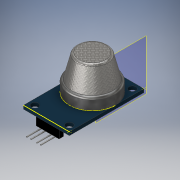
# Autodesk Inventor part: CO2_Sensor
Saved by Autodesk Inventor 2017.2 (Build 212223000, 223)
## iProperties
Created: 2017-03-02
Part Number: CO2_Sensor
Material: Generic
Document SubType Name: Modeling
Designer: prosp
Density: 1 g/cm^3
Appearance: Default
Author: prosp
Autodesk Inventor part; units mm, degrees
ref_plane "YZ Plane" through (0, 0, 0) normal (1, 0, 0) x (0, 1, 0)
ref_plane "XZ Plane" through (0, 0, 0) normal (0, 1, 0) x (-1, 0, 0)
ref_plane "XY Plane" through (0, 0, 0) normal (0, 0, 1) x (1, 0, 0)
sketch "Sketch1" plane through (0, 0, 0) normal (0, 1, 0) x (-1, 0, 0)
  line L0 (10, 16.25) -> (10, -16.25)
  line L1 (10, -16.25) -> (-10, -16.25)
  line L2 (-10, -16.25) -> (-10, 16.25)
  line L3 (-10, 16.25) -> (10, 16.25)
  line L4 (10, 16.25) -> (-10, -16.25) construction
  line L5 (10, -16.25) -> (-10, 16.25) construction
  point P0 (0, 0)
  dimension "d0" = 32.5
  dimension "d1" = 20
  constraints: 12 end point, 2 midpoint, 2 parallel, 1 perpendicular, 1 vertical
  measures "d0" distance of L0.start L0.end
  measures "d1" distance of L0.end L1.end
extrude "Extrusion1" add sketch "Sketch1" along normal blind 1.5
sketch "Sketch2" plane through (0, 1.5, 0) normal (0, 1, 0) x (1, 0, 0)
  line L0 (-10, -16.25) -> (10, -16.25) projected
  point P0 (0, 0)
sketch "Sketch3" plane through (0, 1.5, 0) normal (0, 1, 0) x (1, 0, 0)
  line L0 (-10, -16.25) -> (10, -16.25) projected
  circle A0 centre (0, 3.75) radius 10
  point P0 (0, 0)
  dimension "d7" = 20
  constraints: 1 centre point
  measures "d7" diameter of A0
extrude "Extrusion2" add sketch "Sketch3" along normal blind 5
sketch "Sketch4" plane through (0, 1.5, 0) normal (0, 1, 0) x (1, 0, 0)
  arc A0 (-10, 3.75) -> (10, 3.75) centre (0, 3.75) ccw projected
  point P0 (0, 0)
  point P1 (10, -16.25)
  point P2 (10, 16.25)
fillet "Fillet1" radius 1 1 edges at (-10, 6.5, -3.75)
ref_plane "Work Plane6" through (0, 0, -16.25) normal (-1, 0, 0) x (0, 0, 1)
sketch "Sketch8" plane through (0, 0, -16.25) normal (-1, 0, 0) x (0, 0, 1)
  line L0 (3.5, 6.5) -> (21.5, 6.5) projected
  line L1 (12.5, 6.5) -> (20.5, 6.5)
  line L2 (12.5, 16.5) -> (19, 16.5)
  line L3 (19, 16.5) -> (21.5, 6.5)
  line L4 (12.5, 16.5) -> (12.5, 6.5)
  point P0 (16.25, 0)
  dimension "d20" = 8
  dimension "d21" = 10
  dimension "d22" = 6.5
  constraints: 8 end point, 1 midpoint, 1 point on line, 1 vertical
  measures "d20" distance of L1.start L1.end
  measures "d21" distance of L1.start L2.start
  measures "d22" distance of L2.start L2.end
revolve "Revolution1" add sketch "Sketch8" angle 360 about axis through (0, 16.5, -3.75) along (0, -1, 0)
fillet "Fillet2" radius 1 1 edges at (0, 16.5, -10.25)
sketch "Sketch9" plane through (0, 0, 0) normal (0, -1, 0) x (1, 0, 0)
  circle A0 centre (4.5854, -5.8245) radius 0.25
  circle A1 centre (4.3074, -0.1027) radius 0.25
  circle A2 centre (-1.2201, 1.4011) radius 0.25
  circle A3 centre (-4.3585, -3.3913) radius 0.25
  circle A4 centre (-0.7705, -7.8569) radius 0.25
  point P0 (0, 0)
  point P1 (0.5087, -3.1549)
  dimension "d26" = 0.5
  dimension "d30" = 360
  constraints: 5 centre point, 11 other
  measures "d26" diameter of A0
extrude "Extrusion3" add sketch "Sketch9" along normal blind 5
sketch "Sketch10" plane through (0, 0, 0) normal (0, -1, 0) x (1, 0, 0)
  line L0 (-10, 16.25) -> (-10, -16.25) projected
  line L1 (-10, -16.25) -> (10, -16.25) projected
  circle A0 centre (7.5, -13.75) radius 1.5
  circle A1 centre (-7.5, 13.7454) radius 1.5
  circle A2 centre (7.5, 13.75) radius 1.5
  line L2 (10, -16.25) -> (10, 16.25) projected
  circle A3 centre (-7.5, -13.75) radius 1.5
  point P0 (0, 0)
  dimension "d51" = 3
  constraints: 4 centre point
  measures "d51" diameter of A3
sketch "Sketch11" plane through (0, 0, 0) normal (0, -1, 0) x (1, 0, 0)
  point P0 (0, 0)
hole "Hole1" at (-7.5, 0, 13.7454) at (7.5, 0, 13.75) at (7.5, 0, -13.75) at (-7.5, 0, -13.75) direction (0, 1, 0) diameter 3 end through all
sketch "Sketch12" plane through (0, 0, 0) normal (0, -1, 0) x (1, 0, 0)
  line L0 (-10, 16.25) -> (10, 16.25) projected
  line L1 (5, 15.75) -> (-5, 15.75)
  line L2 (-5, 15.75) -> (-5, 13.75)
  line L3 (-5, 13.75) -> (5, 13.75)
  line L4 (5, 13.75) -> (5, 15.75)
  point P0 (0, 0)
  constraints: 8 end point, 2 parallel, 1 horizontal, 1 perpendicular
extrude "Extrusion4" add sketch "Sketch12" along normal blind 4
sketch "Sketch13" plane through (-5, 0, 15.75) normal (0, 0, 1) x (1, 0, 0)
  circle A0 centre (6.3322, -4.25) radius 0.25
  circle A1 centre (7.977, -4.25) radius 0.25
  circle A2 centre (3.7048, -4.25) radius 0.25
  circle A3 centre (1.889, -4.25) radius 0.25
  line L0 (10, -4) -> (0, -4) projected
  point P0 (5, 0)
  dimension "d64" = 0.5
  dimension "d65" = 0.5
  dimension "d66" = 0.5
  dimension "d67" = 0.5
  constraints: 4 centre point, 4 tangent
  measures "d64" diameter of A0
  measures "d65" diameter of A1
  measures "d66" diameter of A2
  measures "d67" diameter of A3
extrude "Extrusion5" add sketch "Sketch13" along normal blind 6 and the other way blind 1
body "Solid1"
